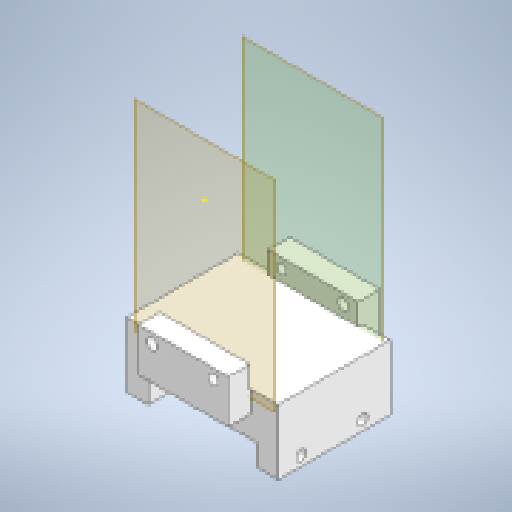
# Autodesk Inventor part: 39
Saved by Autodesk Inventor 2024.3 (Build 283343000, 343)
## iProperties
Created: 2024-09-07
Part Number: 39
Material: LCP 플라스틱
Document SubType Name: Modeling
Designer: 구지현
Density: 1.626 g/cm^3
Appearance: 매끄러움 - 흰색
Mass: 12.8344 g
Surface Area: 38.5805 cm^2
Volume: 7.89322 cm^3
Author: 구지현
Autodesk Inventor part; units mm, degrees
ref_plane "YZ Plane" through (0, 0, 0) normal (1, 0, 0) x (0, 1, 0)
ref_plane "XZ Plane" through (0, 0, 0) normal (0, 1, 0) x (-1, 0, 0)
ref_plane "XY Plane" through (0, 0, 0) normal (0, 0, 1) x (1, 0, 0)
ref_plane "작업 평면1" through (0, 0, 0) normal (0, 0, 1) x (1, 0, 0)
sketch "스케치1" plane through (0, 0, 0) normal (0, 0, 1) x (1, 0, 0)
  line L0 (-12.7, 12) -> (-9.2, 12) projected
  line L1 (-12.7, 12) -> (-17.8, 6) projected
  line L2 (-17.8, 6) -> (-17.8, -32.6) projected
  line L3 (-17.8, -32.6) -> (-12.7, -38.6) projected
  line L4 (-12.7, -38.6) -> (12.7, -38.6) projected
  line L5 (12.7, -38.6) -> (17.8, -32.6) projected
  line L6 (17.8, -32.6) -> (17.8, 6) projected
  line L7 (17.8, 6) -> (12.7, 12) projected
  line L8 (9.2, 12) -> (12.7, 12) projected
  arc A0 (12.2, 9) -> (9.2, 12) centre (9.2, 9) ccw projected
  line L9 (12.2, -30) -> (12.2, 9) projected
  arc A1 (9.2, -33) -> (12.2, -30) centre (9.2, -30) ccw projected
  line L10 (-9.2, -33) -> (9.2, -33) projected
  arc A2 (-12.2, -30) -> (-9.2, -33) centre (-9.2, -30) ccw projected
  line L11 (-12.2, 9) -> (-12.2, -30) projected
  arc A3 (-9.2, 12) -> (-12.2, 9) centre (-9.2, 9) ccw projected
  circle A4 centre (-15, 4.5) radius 1.35 projected
  circle A5 centre (-15, -12.5) radius 1.35 projected
  circle A6 centre (-8.5, -35.8) radius 1.35 projected
  circle A7 centre (15, 4.5) radius 1.35 projected
  circle A8 centre (15, -12.5) radius 1.35 projected
  circle A9 centre (8.5, -35.8) radius 1.35 projected
  circle A10 centre (-15, -29.5) radius 1.35 projected
  circle A11 centre (15, -29.5) radius 1.35 projected
  arc A12 (9.2, -33.1) -> (12.3, -30) centre (9.2, -30) ccw
  line L12 (12.3, -30) -> (12.3, 9)
  arc A13 (12.3, 9) -> (10.2954, 11.9) centre (9.2, 9) ccw
  line L13 (10.2954, 11.9) -> (12.6538, 11.9)
  line L14 (12.6538, 11.9) -> (17.7, 5.9632)
  line L15 (17.7, 5.9632) -> (17.7, -32.5632)
  line L16 (17.7, -32.5632) -> (12.6538, -38.5)
  line L17 (12.6538, -38.5) -> (-12.6538, -38.5)
  line L18 (-12.6538, -38.5) -> (-17.7, -32.5632)
  line L19 (-17.7, -32.5632) -> (-17.7, 5.9632)
  line L20 (-17.7, 5.9632) -> (-12.6538, 11.9)
  line L21 (-12.6538, 11.9) -> (-10.2954, 11.9)
  arc A14 (-10.2954, 11.9) -> (-12.3, 9) centre (-9.2, 9) ccw
  line L22 (-12.3, 9) -> (-12.3, -30)
  arc A15 (-12.3, -30) -> (-9.2, -33.1) centre (-9.2, -30) ccw
  line L23 (-9.2, -33.1) -> (9.2, -33.1)
  circle A16 centre (-8.5, -35.8) radius 1.45
  circle A17 centre (8.5, -35.8) radius 1.45
  line L24 (12.6538, -33.1) -> (-12.3462, -33.1)
  line L25 (-12.3462, -33.1) -> (-12.3462, -39.1)
  line L26 (-12.3462, -39.1) -> (12.6538, -39.1)
  line L27 (12.6538, -39.1) -> (12.6538, -33.1)
  point P0 (0, 0)
  point P1 (9.2, -33.1)
  point P2 (-9.2, -33.1)
  dimension "d0" = 0.1
  dimension "d1" = 0.1
  dimension "d2" = 0.1
  dimension "d3" = 25
  dimension "d4" = 6
  constraints: 32 end point, 8 point on circle, 6 centre point, 2 parallel, 1 horizontal, 1 perpendicular, 15 other
  measures "d0" distance between parallel lines of L10 L23
  measures "d1" radial gap between concentric circles of A6 A16
  measures "d2" radial gap between concentric circles of A9 A17
  measures "d3" distance of L26.end L25.end
  measures "d4" distance of L25.end L24.end
extrude "돌출1" add sketch "스케치1" along normal blind 6 contours L25 L17 L27 L4 | L4 L27 L26 L25 | L25 L24 L23 L27 L17
ref_plane "작업 평면2" through (0, 0, -30) normal (0, 0, -1) x (-1, 0, 0)
sketch "스케치2" plane through (0, 0, -30) normal (0, 0, -1) x (-1, 0, 0)
  line L0 (-12.6538, -33.1) -> (12.3462, -33.1) projected
  line L1 (12.3462, -33.1) -> (12.3462, -39.1) projected
  line L2 (12.3462, -39.1) -> (-12.6538, -39.1) projected
  line L3 (-12.6538, -39.1) -> (-12.6538, -33.1) projected
  circle A0 centre (8.5, -35.8) radius 1.45 projected
  circle A1 centre (-8.5, -35.8) radius 1.45 projected
  point P0 (0, 0)
extrude "돌출2" add sketch "스케치2" along normal blind 6
sketch "스케치3" plane through (-12.3462, -39.1, -30) normal (0, -1, 0) x (1, 0, 0)
  line L0 (0, 30) -> (25, 30) projected
  line L1 (25, 30) -> (25, 36) projected
  line L2 (0, 36) -> (25, 36) projected
  line L3 (0, 30) -> (0, 36) projected
  line L4 (25, 0) -> (0, 0) projected
  line L5 (0, 0) -> (0, -6) projected
  line L6 (25, -6) -> (0, -6) projected
  line L7 (25, 0) -> (25, -6) projected
  line L8 (25, 36) -> (0, 36)
  line L9 (0, 36) -> (0, -6)
  line L10 (0, -6) -> (25, -6)
  line L11 (25, -6) -> (25, 36)
  point P0 (12.3462, 30)
  constraints: 8 end point, 2 parallel, 1 horizontal, 1 perpendicular
extrude "돌출3" add sketch "스케치3" along normal blind 6
sketch "스케치5" plane through (-12.3462, -45.1, -30) normal (0, -1, 0) x (1, 0, 0)
  circle A0 centre (11.5825, 20.4065) radius 1.6 projected
  line L0 (26.6325, 7.8369) -> (26.6325, 32.8369) projected
  line L1 (-3.3675, 32.8369) -> (26.6325, 32.8369) projected
  line L2 (-3.3675, 32.8369) -> (-3.3675, 7.8369) projected
  line L3 (26.6325, 7.8369) -> (-3.3675, 7.8369) projected
  line L4 (-3.3675, 7.8369) -> (-3.3675, 32.8369) projected
  line L5 (-3.3675, 32.8369) -> (-9.3675, 32.8369) projected
  line L6 (-9.3675, 7.8369) -> (-9.3675, 32.8369) projected
  line L7 (-3.3675, 7.8369) -> (-9.3675, 7.8369) projected
  line L8 (26.6325, 32.8369) -> (26.6325, 7.8369) projected
  line L9 (26.6325, 7.8369) -> (32.6325, 7.8369) projected
  line L10 (32.6325, 32.8369) -> (32.6325, 7.8369) projected
  line L11 (26.6325, 32.8369) -> (32.6325, 32.8369) projected
  line L12 (32.6325, 7.8369) -> (-9.3675, 7.8369)
  line L13 (-9.3675, 7.8369) -> (-9.3675, 1.8369)
  line L14 (-9.3675, 1.8369) -> (32.6325, 1.8369)
  line L15 (32.6325, 1.8369) -> (32.6325, 7.8369)
  line L16 (26.6325, 7.8369) -> (26.6325, 1.8369)
  line L17 (-3.3675, 7.8369) -> (-3.3675, 1.8369)
  line L18 (32.6325, 1.8369) -> (-9.3675, 1.8369)
  line L19 (-9.3675, 1.8369) -> (-9.3675, -1.1631)
  line L20 (-9.3675, -1.1631) -> (32.6325, -1.1631)
  line L21 (32.6325, -1.1631) -> (32.6325, 1.8369)
  line L22 (-9.3675, 32.8369) -> (32.6325, 32.8369)
  line L23 (32.6325, 32.8369) -> (32.6325, 29.8369)
  line L24 (32.6325, 29.8369) -> (-9.3675, 29.8369)
  line L25 (-9.3675, 29.8369) -> (-9.3675, 32.8369)
  point P0 (12.3462, 30)
  point P1 (-9.3675, 29.8369)
  dimension "d18" = 6
  dimension "d24" = 3
  dimension "d25" = 3
  constraints: 28 end point, 6 parallel, 5 perpendicular, 3 horizontal, 3 point on line
  measures "d18" distance of L13.end L12.end
  measures "d24" distance of L19.end L18.end
  measures "d25" distance of L22.end L23.end
extrude "돌출5" add sketch "스케치5" along normal blind 6 contours A0 | L3 L2 L24 L0 | L16 L14 L17 L3 | L0 L24 L10 L9 | L9 L15 L14 L16 | L7 L6 L24 L2 | L17 L14 L13 L7 | L14 L21 L20 L19
sketch "스케치6" plane through (-12.3462, -51.1, -30) normal (0, -1, 0) x (1, 0, 0)
  line L0 (-3.3675, 7.8369) -> (-3.3675, 32.8369) projected
  line L1 (-3.3675, 32.8369) -> (-9.3675, 32.8369) projected
  line L2 (-9.3675, 7.8369) -> (-9.3675, 32.8369) projected
  line L3 (-3.3675, 7.8369) -> (-9.3675, 7.8369) projected
  line L4 (26.6325, 32.8369) -> (26.6325, 7.8369) construction
  line L5 (26.6325, 7.8369) -> (32.6325, 7.8369) construction
  line L6 (32.6325, 32.8369) -> (32.6325, 7.8369) construction
  line L7 (26.6325, 32.8369) -> (32.6325, 32.8369) construction
  line L8 (26.6325, 32.8369) -> (26.6325, 7.8369) projected
  line L9 (26.6325, 7.8369) -> (32.6325, 7.8369) projected
  line L10 (32.6325, 32.8369) -> (32.6325, 7.8369) projected
  line L11 (26.6325, 32.8369) -> (32.6325, 32.8369) projected
  line L12 (32.6325, -1.1631) -> (32.6325, 29.8369) projected
  line L13 (32.6325, 29.8369) -> (-9.3675, 29.8369) projected
  line L14 (-9.3675, 29.8369) -> (-9.3675, -1.1631) projected
  line L15 (-9.3675, -1.1631) -> (32.6325, -1.1631) projected
  line L16 (-9.3675, 29.8369) -> (-9.3675, -1.1631) projected
  line L17 (-3.3675, 7.8369) -> (-9.3675, 7.8369)
  line L18 (-9.3675, 7.8369) -> (-9.3675, -1.1631)
  line L19 (-9.3675, -1.1631) -> (-3.3675, -1.1631)
  line L20 (-3.3675, -1.1631) -> (-3.3675, 7.8369)
  line L21 (26.6325, 7.8369) -> (32.6325, 7.8369)
  line L22 (32.6325, 7.8369) -> (32.6325, -1.1631)
  line L23 (32.6325, -1.1631) -> (26.6325, -1.1631)
  line L24 (26.6325, -1.1631) -> (26.6325, 7.8369)
  point P0 (-3.3675, 29.8369)
  point P1 (26.6325, 29.8369)
  point P2 (-3.3675, -1.1631)
  constraints: 16 end point, 4 parallel, 2 horizontal, 2 perpendicular
extrude "돌출6" add sketch "스케치6" along normal blind 6 contours L3 L2 L13 L0 | L20 L15 L14 L3 | L13 L10 L9 L8 | L24 L9 L12 L15
sketch "스케치8" plane through (20.2862, -45.1, -0.1631) normal (1, 0, 0) x (0, 0, -1)
  line L0 (27.5869, -57.1) -> (24.0869, -57.1) projected
  line L1 (27.5869, -57.1) -> (32.6869, -51.1) projected
  line L2 (32.6869, -51.1) -> (32.6869, -12.5) projected
  line L3 (32.6869, -12.5) -> (27.5869, -6.5) projected
  line L4 (27.5869, -6.5) -> (2.1869, -6.5) projected
  line L5 (2.1869, -6.5) -> (-2.9131, -12.5) projected
  line L6 (-2.9131, -12.5) -> (-2.9131, -51.1) projected
  line L7 (-2.9131, -51.1) -> (2.1869, -57.1) projected
  line L8 (5.6869, -57.1) -> (2.1869, -57.1) projected
  arc A0 (2.6869, -54.1) -> (5.6869, -57.1) centre (5.6869, -54.1) ccw projected
  line L9 (2.6869, -15.1) -> (2.6869, -54.1) projected
  arc A1 (5.6869, -12.1) -> (2.6869, -15.1) centre (5.6869, -15.1) ccw projected
  line L10 (24.0869, -12.1) -> (5.6869, -12.1) projected
  arc A2 (27.0869, -15.1) -> (24.0869, -12.1) centre (24.0869, -15.1) ccw projected
  line L11 (27.0869, -54.1) -> (27.0869, -15.1) projected
  arc A3 (24.0869, -57.1) -> (27.0869, -54.1) centre (24.0869, -54.1) ccw projected
  circle A4 centre (29.8869, -49.6) radius 1.35 projected
  circle A5 centre (29.8869, -32.6) radius 1.35 projected
  circle A6 centre (23.3869, -9.3) radius 1.35 projected
  circle A7 centre (-0.1131, -49.6) radius 1.35 projected
  circle A8 centre (-0.1131, -32.6) radius 1.35 projected
  circle A9 centre (6.3869, -9.3) radius 1.35 projected
  circle A10 centre (29.8869, -15.6) radius 1.35 projected
  circle A11 centre (-0.1131, -15.6) radius 1.35 projected
  circle A12 centre (6.3869, -9.3) radius 1.35 projected
  circle A13 centre (6.3869, -9.3) radius 1.45
  circle A14 centre (23.3869, -9.3) radius 1.45
  point P0 (-0.1631, 45.1)
  dimension "d26" = 0.1
  dimension "d27" = 0.1
  constraints: 2 centre point
  measures "d26" radial gap between concentric circles of A9 A13
  measures "d27" radial gap between concentric circles of A6 A14
extrude "돌출8" cut sketch "스케치8" against normal blind 50 contours A6 | A9 | A13 | A14
sketch "스케치9" plane through (-12.3462, -45.1, -30) normal (0, 1, 0) x (1, 0, 0)
  line L0 (25, 1.1631) -> (25, -29.8369) projected
  line L1 (32.6325, -29.8369) -> (25, -29.8369) projected
  line L2 (32.6325, 1.1631) -> (32.6325, -29.8369) projected
  line L3 (25, 1.1631) -> (32.6325, 1.1631) projected
  line L4 (0, -29.8369) -> (0, 1.1631) projected
  line L5 (-9.3675, 1.1631) -> (0, 1.1631) projected
  line L6 (-9.3675, -29.8369) -> (-9.3675, 1.1631) projected
  line L7 (0, -29.8369) -> (-9.3675, -29.8369) projected
  point P0 (12.3462, -30)
extrude "돌출9" add sketch "스케치9" along normal blind 6
sketch "스케치10" plane through (-21.7138, -45.1, -0.1631) normal (0, 0, 1) x (1, 0, 0)
  line L0 (9.3675, 12) -> (9.3675, 0) projected
  line L1 (9.3675, 12) -> (34.3675, 12) projected
  line L2 (34.3675, 12) -> (34.3675, 0) projected
  line L3 (9.3675, 0) -> (34.3675, 0) projected
  circle A0 centre (30.2138, 9.3) radius 1.45 projected
  circle A1 centre (13.2138, 9.3) radius 1.45 projected
  line L4 (34.3675, 0) -> (9.3675, 0) projected
  line L5 (34.3675, 6) -> (34.3675, 0) projected
  line L6 (42, 6) -> (34.3675, 6) projected
  line L7 (42, -12) -> (42, 6) projected
  line L8 (36, -12) -> (42, -12) projected
  line L9 (36, -6) -> (36, -12) projected
  line L10 (6, -6) -> (36, -6) projected
  line L11 (6, -6) -> (6, -12) projected
  line L12 (0, -12) -> (6, -12) projected
  line L13 (0, 6) -> (0, -12) projected
  line L14 (9.3675, 6) -> (0, 6) projected
  line L15 (9.3675, 0) -> (9.3675, 6) projected
  line L16 (6, -6) -> (6, 4.4236)
  line L17 (36, -6) -> (6, -6) projected
  line L18 (36, -6) -> (36, 5.3756)
  line L19 (36, -6) -> (6, -6)
  line L20 (6, -6) -> (6, 0)
  line L21 (6, 0) -> (36, 0)
  line L22 (36, 0) -> (36, -6)
  point P0 (21.7138, 45.1)
  point P1 (36, 0)
  constraints: 12 end point, 2 parallel, 2 vertical, 1 horizontal, 1 perpendicular, 1 point on line
extrude "돌출10" cut sketch "스케치10" against normal blind 50 contours L3 L21 L18 L10 L16
sketch "스케치11" plane through (12.6538, -33.1, -30) normal (1, 0, 0) x (0, 0, -1)
  line L0 (0, -6) -> (1.1631, -6) projected
  line L1 (1.1631, -6) -> (1.1631, -12) projected
  line L2 (6, -12) -> (1.1631, -12) projected
  line L3 (6, 0) -> (6, -12) projected
  line L4 (0, 0) -> (6, 0) projected
  line L5 (0, 0) -> (0, -6) projected
  line L6 (-29.8369, -12) -> (-29.8369, -6) projected
  line L7 (-29.8369, -6) -> (-30, -6) projected
  line L8 (-30, -6) -> (-30, 0) projected
  line L9 (-30, 0) -> (-36, 0) projected
  line L10 (-36, 0) -> (-36, -12) projected
  line L11 (-29.8369, -12) -> (-36, -12) projected
  line L12 (-29.8369, -12) -> (-29.8369, -6) projected
  line L13 (-29.8369, -6) -> (-30, -6) projected
  line L14 (-30, -6) -> (-30, 0) projected
  line L15 (-30, 0) -> (-36, 0) projected
  line L16 (-36, 0) -> (-36, -12) projected
  line L17 (-29.8369, -12) -> (-36, -12) projected
  line L18 (0, -6) -> (1.1631, -6) projected
  line L19 (1.1631, -6) -> (1.1631, -12) projected
  line L20 (6, -12) -> (1.1631, -12) projected
  line L21 (6, 0) -> (6, -12) projected
  line L22 (0, 0) -> (6, 0) projected
  line L23 (0, 0) -> (0, -6) projected
  point P0 (-30, 33.1)
extrude "돌출11" cut sketch "스케치11" against normal blind 50
sketch "스케치12" plane through (20.2862, -39.1, -0.1631) normal (1, 0, 0) x (0, 0, -1)
  line L0 (29.8369, -5.5) -> (29.8369, 0.5) projected
  line L1 (4.3369, -5.5) -> (4.3369, -0.375) projected
  line L2 (29.8369, 0.5) -> (29.8369, -18)
  line L3 (0, -18) -> (31, -18) projected
  circle A0 centre (6.3869, -15.3) radius 1.45 projected
  circle A1 centre (23.3869, -15.3) radius 1.45 projected
  line L4 (0, 0) -> (0, -18) projected
  line L5 (31, -18) -> (0, -18) projected
  line L6 (31, -18) -> (31, 0) projected
  line L7 (0, 0) -> (31, 0) projected
  point P0 (-0.1631, 39.1)
  point P1 (29.8369, 0)
  constraints: 2 end point, 1 point on line, 1 vertical, 1 other
extrude "돌출12" cut sketch "스케치12" against normal blind 50 contours L0 L7 L6 L3 L2
sketch "스케치13" plane through (20.2862, -57.1, -0.1631) normal (1, 0, 0) x (0, 0, -1)
  line L0 (29.8369, 12.5) -> (29.8369, 18.5) projected
  line L1 (29.8369, 0) -> (29.8369, 18) projected
  line L2 (4.3369, 12.5) -> (4.3369, 17.625) projected
  line L3 (-0.1631, 12.5) -> (-0.1631, 18.5) projected
  line L4 (0, 18) -> (0, 0) projected
  line L5 (4.3369, 12.5) -> (4.3369, 17.625) projected
  line L6 (4.3369, 12.5) -> (4.3369, 17.625) projected
  line L7 (4.3369, 12.5) -> (4.3369, 17.625) projected
  line L8 (4.3369, 18.1) -> (25.3369, 18.1) projected
  line L9 (4.4369, 18.5) -> (4.4369, 23.625)
  line L10 (4.3369, 18) -> (25.3369, 18)
  line L11 (25.3369, 12.5) -> (25.3369, 17.625) projected
  line L12 (25.2369, 18.5) -> (25.2369, 23.625)
  line L13 (4.4369, 18.5) -> (4.4369, 18)
  line L14 (29.8369, 18) -> (0, 18) projected
  line L15 (4.4369, 18) -> (4.4369, 12.4)
  line L16 (4.4369, 12.4) -> (0, 12.4)
  line L17 (25.2369, 18.5) -> (25.2369, 18)
  line L18 (25.2369, 18) -> (25.2369, 12.4)
  line L19 (25.2369, 12.4) -> (29.8369, 12.4)
  point P0 (-0.1631, 57.1)
  dimension "d38" = 0.1
  dimension "d39" = 0.1
  dimension "d40" = 0.1
  dimension "d41" = 5.6
  dimension "d42" = 5.6
  constraints: 18 end point, 6 point on line, 3 parallel, 3 perpendicular, 1 vertical
  measures "d38" distance between parallel lines of L2 L9
  measures "d39" distance between parallel lines of L8 L10
  measures "d40" distance between parallel lines of L11 L12
  measures "d41" distance of L13.end L15.end
  measures "d42" distance of L17.end L18.end
extrude "돌출13" cut sketch "스케치13" against normal blind 50 contours L1 L19 L18 L10 L14 L0 | L15 L16 L4 L14 L10
sketch "스케치14" plane through (20.2862, -44.7, -4.6) normal (0, 0, 1) x (1, 0, 0)
  line L0 (-32.9862, 50.7) -> (-29.4862, 50.7) projected
  line L1 (-32.9862, 50.7) -> (-38.0862, 44.7) projected
  line L2 (-38.0862, 44.7) -> (-38.0862, 6.1) projected
  line L3 (-38.0862, 6.1) -> (-32.9862, 0.1) projected
  line L4 (-32.9862, 0.1) -> (-7.5862, 0.1) projected
  line L5 (-7.5862, 0.1) -> (-2.4862, 6.1) projected
  line L6 (-2.4862, 6.1) -> (-2.4862, 44.7) projected
  line L7 (-2.4862, 44.7) -> (-7.5862, 50.7) projected
  line L8 (-11.0862, 50.7) -> (-7.5862, 50.7) projected
  arc A0 (-8.0862, 47.7) -> (-11.0862, 50.7) centre (-11.0862, 47.7) ccw projected
  line L9 (-8.0862, 8.7) -> (-8.0862, 47.7) projected
  arc A1 (-11.0862, 5.7) -> (-8.0862, 8.7) centre (-11.0862, 8.7) ccw projected
  line L10 (-29.4862, 5.7) -> (-11.0862, 5.7) projected
  arc A2 (-32.4862, 8.7) -> (-29.4862, 5.7) centre (-29.4862, 8.7) ccw projected
  line L11 (-32.4862, 47.7) -> (-32.4862, 8.7) projected
  arc A3 (-29.4862, 50.7) -> (-32.4862, 47.7) centre (-29.4862, 47.7) ccw projected
  circle A4 centre (-35.2862, 43.2) radius 1.35 projected
  circle A5 centre (-35.2862, 26.2) radius 1.35 projected
  circle A6 centre (-28.7862, 2.9) radius 1.35 projected
  circle A7 centre (-5.2862, 43.2) radius 1.35 projected
  circle A8 centre (-5.2862, 26.2) radius 1.35 projected
  circle A9 centre (-11.7862, 2.9) radius 1.35 projected
  circle A10 centre (-35.2862, 9.2) radius 1.35 projected
  circle A11 centre (-5.2862, 9.2) radius 1.35 projected
  circle A12 centre (-11.7862, 2.9) radius 1.45
  circle A13 centre (-28.7862, 2.9) radius 1.45
  dimension "d48" = 0.1
  dimension "d49" = 0.1
  constraints: 2 centre point
  measures "d48" radial gap between concentric circles of A9 A12
  measures "d49" radial gap between concentric circles of A6 A13
sketch "스케치15" plane through (-15.7138, -45.1, -0.1631) normal (0, 0, 1) x (1, 0, 0)
  line L0 (36, 0.4) -> (-6, 0.4) projected
  line L1 (-6, 0.4) -> (-6, -12) projected
  line L2 (0, -12) -> (-6, -12) projected
  line L3 (0, -12) -> (0, 0) projected
  line L4 (30, 0) -> (0, 0) projected
  line L5 (30, 0) -> (30, -12) projected
  line L6 (36, -12) -> (30, -12) projected
  line L7 (36, 0.4) -> (36, -12) projected
  line L8 (-6, 0.4) -> (-6, -12) projected
  line L9 (36, 0.4) -> (-6, 0.4)
  line L10 (-6, 0.4) -> (-6, -5.6)
  line L11 (-6, -5.6) -> (36, -5.6)
  line L12 (36, -5.6) -> (36, 0.4)
  point P0 (15.7138, 45.1)
  point P1 (36, -5.6)
  point P2 (-6, -5.6)
  dimension "d45" = 6
  constraints: 8 end point, 2 parallel, 1 horizontal, 1 perpendicular, 1 point on line
  measures "d45" distance of L10.end L9.end
extrude "돌출14" add sketch "스케치15" against normal blind 29.837 contours L7 L11 L5 L4 L3 L1 L0 | L11 L3 L4 L5
extrude "돌출15" cut sketch "스케치14" against normal blind 29.837 contours A6 | A9 | A12 | A13
